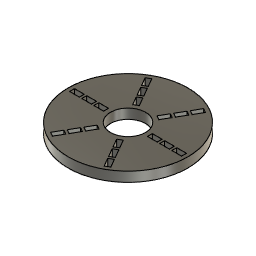
ex49 (Autodesk Fusion 360 design; units mm, degrees)
Autodesk Fusion 360 part; units mm, degrees
sketch "Sketch1" plane through (0, 0, 0) normal (0, 0, 1) x (1, 0, 0)
  circle A0 centre (0, 0) radius 122.75
  circle A1 centre (0, 0) radius 36
  line L0 (45, 5) -> (65, 5)
  line L1 (65, 5) -> (65, -5)
  line L2 (65, -5) -> (45, -5)
  line L3 (45, -5) -> (45, 5)
  line L4 (70, -5) -> (70, 5)
  line L5 (70, 5) -> (90, 5)
  line L6 (90, -5) -> (70, -5)
  line L7 (90, 5) -> (90, -5)
  line L8 (95, -5) -> (95, 5)
  line L9 (95, 5) -> (115, 5)
  line L10 (115, -5) -> (95, -5)
  line L11 (115, 5) -> (115, -5)
  line L12 (40.6699, 80.4423) -> (49.3301, 75.4423)
  line L13 (18.1699, 41.4711) -> (28.1699, 58.7917)
  line L14 (49.3301, 75.4423) -> (39.3301, 58.1218)
  line L15 (28.1699, 58.7917) -> (36.8301, 53.7917)
  line L16 (30.6699, 63.1218) -> (40.6699, 80.4423)
  line L17 (53.1699, 102.0929) -> (61.8301, 97.0929)
  line L18 (51.8301, 79.7724) -> (43.1699, 84.7724)
  line L19 (43.1699, 84.7724) -> (53.1699, 102.0929)
  line L20 (61.8301, 97.0929) -> (51.8301, 79.7724)
  line L21 (26.8301, 36.4711) -> (18.1699, 41.4711)
  line L22 (39.3301, 58.1218) -> (30.6699, 63.1218)
  line L23 (36.8301, 53.7917) -> (26.8301, 36.4711)
  line L24 (-49.3301, 75.4423) -> (-40.6699, 80.4423)
  line L25 (-26.8301, 36.4711) -> (-36.8301, 53.7917)
  line L26 (-40.6699, 80.4423) -> (-30.6699, 63.1218)
  line L27 (-36.8301, 53.7917) -> (-28.1699, 58.7917)
  line L28 (-39.3301, 58.1218) -> (-49.3301, 75.4423)
  line L29 (-61.8301, 97.0929) -> (-53.1699, 102.0929)
  line L30 (-43.1699, 84.7724) -> (-51.8301, 79.7724)
  line L31 (-51.8301, 79.7724) -> (-61.8301, 97.0929)
  line L32 (-53.1699, 102.0929) -> (-43.1699, 84.7724)
  line L33 (-18.1699, 41.4711) -> (-26.8301, 36.4711)
  line L34 (-30.6699, 63.1218) -> (-39.3301, 58.1218)
  line L35 (-28.1699, 58.7917) -> (-18.1699, 41.4711)
  line L36 (-90, -5) -> (-90, 5)
  line L37 (-45, -5) -> (-65, -5)
  line L38 (-90, 5) -> (-70, 5)
  line L39 (-65, -5) -> (-65, 5)
  line L40 (-70, -5) -> (-90, -5)
  line L41 (-115, -5) -> (-115, 5)
  line L42 (-95, 5) -> (-95, -5)
  line L43 (-95, -5) -> (-115, -5)
  line L44 (-115, 5) -> (-95, 5)
  line L45 (-45, 5) -> (-45, -5)
  line L46 (-70, 5) -> (-70, -5)
  line L47 (-65, 5) -> (-45, 5)
  line L48 (-40.6699, -80.4423) -> (-49.3301, -75.4423)
  line L49 (-18.1699, -41.4711) -> (-28.1699, -58.7917)
  line L50 (-49.3301, -75.4423) -> (-39.3301, -58.1218)
  line L51 (-28.1699, -58.7917) -> (-36.8301, -53.7917)
  line L52 (-30.6699, -63.1218) -> (-40.6699, -80.4423)
  line L53 (-53.1699, -102.0929) -> (-61.8301, -97.0929)
  line L54 (-51.8301, -79.7724) -> (-43.1699, -84.7724)
  line L55 (-43.1699, -84.7724) -> (-53.1699, -102.0929)
  line L56 (-61.8301, -97.0929) -> (-51.8301, -79.7724)
  line L57 (-26.8301, -36.4711) -> (-18.1699, -41.4711)
  line L58 (-39.3301, -58.1218) -> (-30.6699, -63.1218)
  line L59 (-36.8301, -53.7917) -> (-26.8301, -36.4711)
  line L60 (49.3301, -75.4423) -> (40.6699, -80.4423)
  line L61 (26.8301, -36.4711) -> (36.8301, -53.7917)
  line L62 (40.6699, -80.4423) -> (30.6699, -63.1218)
  line L63 (36.8301, -53.7917) -> (28.1699, -58.7917)
  line L64 (39.3301, -58.1218) -> (49.3301, -75.4423)
  line L65 (61.8301, -97.0929) -> (53.1699, -102.0929)
  line L66 (43.1699, -84.7724) -> (51.8301, -79.7724)
  line L67 (51.8301, -79.7724) -> (61.8301, -97.0929)
  line L68 (53.1699, -102.0929) -> (43.1699, -84.7724)
  line L69 (18.1699, -41.4711) -> (26.8301, -36.4711)
  line L70 (30.6699, -63.1218) -> (39.3301, -58.1218)
  line L71 (28.1699, -58.7917) -> (18.1699, -41.4711)
  dimension "d1" = 245.5
  dimension "d2" = 72
  dimension "d4" = 20
  dimension "d5" = 10
  dimension "d6" = 20
  dimension "d7" = 10
  dimension "d8" = 20
  dimension "d9" = 10
  dimension "d11" = 360
  constraint coincident A0.centre A1.centre
  constraint concentric A0 A1
  constraint horizontal L0
  constraint vertical L1
  constraint horizontal L2
  constraint vertical L3
  constraint horizontal L5
  constraint vertical L7
  constraint horizontal L6
  constraint vertical L4
  constraint horizontal L9
  constraint vertical L11
  constraint horizontal L10
  constraint vertical L8
  measures "d1" diameter of A0
  measures "d2" diameter of A1
  measures "d4" distance of L0.start L0.end
  measures "d5" distance of L0.start L2.end
  measures "d6" distance of L4.end L5.end
  measures "d7" distance of L4.end L4.start
  measures "d8" distance of L8.end L9.end
  measures "d9" distance of L8.end L8.start
extrude "Extrude1" add sketch "Sketch1" along normal blind 20
